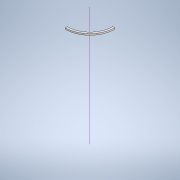
# Autodesk Inventor part: UpperSemiCircle
Saved by Autodesk Inventor 2022 (Build 260153000, 153)
## iProperties
Created: 2022-01-10
Part Number: UpperSemiCircle
Material: Generic
Document SubType Name: Modeling
Designer: Daniel Marquez
Density: 1 g/cm^3
Appearance: Default
Author: Daniel Marquez
Autodesk Inventor part; units mm, degrees
ref_plane "YZ Plane" through (0, 0, 0) normal (1, 0, 0) x (0, 1, 0)
ref_plane "XY Plane" through (0, 0, 0) normal (0, 0, 1) x (1, 0, 0)
ref_plane "Work Plane1" through (0, 2641.6, 0) normal (0, 1, 0) x (-1, 0, 0)
sketch "Sketch1" plane through (0, 2641.6, 0) normal (0, 1, 0) x (-1, 0, 0)
  circle A0 centre (0, 0) radius 609.6
  circle A1 centre (0, 0) radius 660.4
  line L0 (0, 660.4) -> (0, 609.6)
  line L1 (-609.6, 0) -> (-660.4, 0)
  dimension "d1" = 1219.2
  dimension "d2" = 1320.8
  constraints: 4 end point, 4 point on circle, 2 centre point, 2 coincident, 1 perpendicular, 1 vertical
  measures "d1" diameter of A0
  measures "d2" diameter of A1
extrude "Extrusion1" add sketch "Sketch1" along normal blind 38.1 contours A0 L1 A1 L0 picked at (-643.1438, 11.9178)
body "Solid1"
